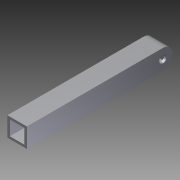
# Autodesk Inventor part: 8 ball pnumatic arm tube
Saved by Autodesk Inventor 2012 (Build 160160000, 160)
## iProperties
Created: 2013-10-08
Part Number: 8 ball pnumatic arm tube
Material: Default
Document SubType Name: Modeling
Designer: Bryce
Density: 1 g/cm^3
Author: Bryce
Autodesk Inventor part; units mm, degrees
ref_plane "YZ Plane" through (0, 0, 0) normal (1, 0, 0) x (0, 1, 0)
ref_plane "XZ Plane" through (0, 0, 0) normal (0, 1, 0) x (-1, 0, 0)
ref_plane "XY Plane" through (0, 0, 0) normal (0, 0, 1) x (1, 0, 0)
sketch "Sketch1" plane through (0, 0, 0) normal (0, 0, 1) x (1, 0, 0)
  line L0 (0, 0) -> (25.4, 0)
  line L1 (25.4, 0) -> (25.4, 25.4)
  line L2 (25.4, 25.4) -> (0, 25.4)
  line L3 (0, 25.4) -> (0, 0)
  line L4 (3.175, 3.175) -> (22.225, 3.175)
  line L5 (22.225, 3.175) -> (22.225, 22.225)
  line L6 (22.225, 22.225) -> (3.175, 22.225)
  line L7 (3.175, 22.225) -> (3.175, 3.175)
  dimension "d0" = 25.4
  dimension "d1" = 25.4
  dimension "d2" = 3.175
  dimension "d3" = 3.175
  dimension "d4" = 3.175
  dimension "d5" = 3.175
  constraints: 16 end point, 4 parallel, 2 horizontal, 2 perpendicular
  measures "d0" distance of L0.start L0.end
  measures "d1" distance of L2.end L0.start
  measures "d2" distance between parallel lines of L0 L4
  measures "d3" distance between parallel lines of L1 L5
  measures "d4" distance between parallel lines of L2 L6
  measures "d5" distance between parallel lines of L3 L7
extrude "Extrusion1" add sketch "Sketch1" along normal blind 190.5
sketch "Sketch2" plane through (25.4, 0, 0) normal (1, 0, 0) x (0, 0, -1)
  line L0 (-190.5, 25.4) -> (-190.5, 0) projected
  line L1 (0, 0) -> (-190.5, 0) projected
  line L2 (0, 0) -> (0, 25.4) projected
  line L3 (0, 25.4) -> (-190.5, 25.4) projected
  circle A0 centre (-12.7, 12.7) radius 4.7625
  arc A1 (-12.7, 0) -> (-12.7, 25.4) centre (-12.7, 12.7) ccw
  dimension "d8" = 9.525
  dimension "d9" = 12.7
  dimension "d10" = 12.7
  constraints: 3 tangent, 2 centre point, 2 point on circle, 2 point on line
  measures "d8" diameter of A0
  measures "d9" distance from line of L3 A0.centre
  measures "d10" distance from line of L2 A0.centre
extrude "Extrusion2" cut sketch "Sketch2" against normal blind 25.4 contours L3 L2 A1 | A1 L2 L1 | A0
equation "\"d2\" = d5"
equation "\"d3\" = d2"
equation "\"d5\" = d4"
equation "\"d10\" = d9"
body "Solid1"
